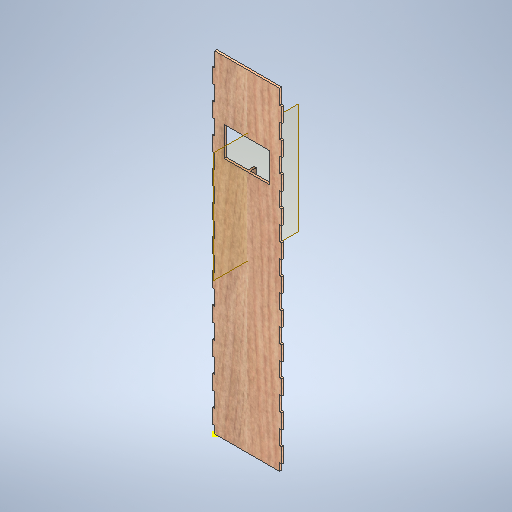
# Autodesk Inventor part: Part4 box
Saved by Autodesk Inventor 2025.3 (Build 293356000, 356)
## iProperties
Created: 2026-04-05
Part Number: Part4 box
Material: Wood (Birch)
Document SubType Name: Modeling
Designer: logien
Density: 0.55 g/cm^3
Appearance: Birch - Natural Polished
Author: logien
Autodesk Inventor part; units mm, degrees
ref_plane "YZ Plane" through (0, 0, 0) normal (1, 0, 0) x (0, 1, 0)
ref_plane "XZ Plane" through (0, 0, 0) normal (0, 1, 0) x (-1, 0, 0)
ref_plane "XY Plane" through (0, 0, 0) normal (0, 0, 1) x (1, 0, 0)
sketch "Sketch1" plane through (0, 0, 0) normal (0, 0, 1) x (1, 0, 0)
  line L0 (0, 0) -> (88, 0)
  line L1 (88, 0) -> (88, 10)
  line L2 (88, 10) -> (91, 10)
  line L3 (91, 10) -> (91, 30)
  line L4 (91, 30) -> (88, 30)
  line L5 (88, 30) -> (88, 50)
  line L6 (88, 50) -> (91, 50)
  line L7 (91, 50) -> (91, 70)
  line L8 (91, 70) -> (88, 70)
  line L9 (88, 70) -> (88, 90)
  line L10 (88, 90) -> (91, 90)
  line L11 (91, 90) -> (91, 110)
  line L12 (91, 110) -> (88, 110)
  line L13 (88, 110) -> (88, 130)
  line L14 (88, 130) -> (91, 130)
  line L15 (91, 130) -> (91, 150)
  line L16 (91, 150) -> (88, 150)
  line L17 (88, 150) -> (88, 170)
  line L18 (88, 170) -> (91, 170)
  line L19 (91, 170) -> (91, 190)
  line L20 (91, 190) -> (88, 190)
  line L21 (88, 190) -> (88, 210)
  line L22 (88, 210) -> (91, 210)
  line L23 (91, 210) -> (91, 230)
  line L24 (91, 230) -> (88, 230)
  line L25 (88, 230) -> (88, 250)
  line L26 (88, 250) -> (91, 250)
  line L27 (91, 250) -> (91, 270)
  line L28 (91, 270) -> (88, 270)
  line L29 (88, 270) -> (88, 290)
  line L30 (88, 290) -> (91, 290)
  line L31 (91, 290) -> (91, 310)
  line L32 (91, 310) -> (88, 310)
  line L33 (88, 310) -> (88, 330)
  line L34 (88, 330) -> (91, 330)
  line L35 (91, 330) -> (91, 350)
  line L36 (91, 350) -> (88, 350)
  line L37 (88, 350) -> (88, 370)
  line L38 (88, 370) -> (91, 370)
  line L39 (91, 370) -> (91, 390)
  line L40 (91, 390) -> (88, 390)
  line L41 (88, 390) -> (88, 410)
  line L42 (88, 410) -> (91, 410)
  line L43 (91, 410) -> (91, 430)
  line L44 (91, 430) -> (88, 430)
  line L45 (44, 0) -> (44, 110) construction
  line L46 (-3, 10) -> (-3, 30)
  line L47 (-3, 30) -> (0, 30)
  line L48 (0, 10) -> (-3, 10)
  line L49 (0, 50) -> (-3, 50)
  line L50 (-3, 50) -> (-3, 70)
  line L51 (0, 70) -> (0, 90)
  line L52 (0, 90) -> (-3, 90)
  line L53 (-3, 90) -> (-3, 110)
  line L54 (-3, 70) -> (0, 70)
  line L55 (-3, 110) -> (0, 110)
  line L56 (0, 110) -> (0, 130)
  line L57 (0, 130) -> (-3, 130)
  line L58 (-3, 130) -> (-3, 150)
  line L59 (-3, 170) -> (-3, 190)
  line L60 (0, 150) -> (0, 170)
  line L61 (0, 170) -> (-3, 170)
  line L62 (-3, 150) -> (0, 150)
  line L63 (0, 190) -> (0, 210)
  line L64 (-3, 190) -> (0, 190)
  line L65 (0, 210) -> (-3, 210)
  line L66 (-3, 210) -> (-3, 230)
  line L67 (-3, 230) -> (0, 230)
  line L68 (0, 230) -> (0, 250)
  line L69 (0, 250) -> (-3, 250)
  line L70 (-3, 250) -> (-3, 270)
  line L71 (-3, 270) -> (0, 270)
  line L72 (0, 270) -> (0, 290)
  line L73 (0, 290) -> (-3, 290)
  line L74 (-3, 290) -> (-3, 310)
  line L75 (-3, 310) -> (0, 310)
  line L76 (0, 310) -> (0, 330)
  line L77 (0, 350) -> (0, 370)
  line L78 (-3, 350) -> (0, 350)
  line L79 (-3, 330) -> (-3, 350)
  line L80 (0, 330) -> (-3, 330)
  line L81 (0, 370) -> (-3, 370)
  line L82 (-3, 370) -> (-3, 390)
  line L83 (-3, 390) -> (0, 390)
  line L84 (0, 390) -> (0, 410)
  line L85 (0, 410) -> (-3, 410)
  line L86 (-3, 410) -> (-3, 430)
  line L87 (-3, 430) -> (0, 430)
  line L88 (0, 430) -> (0, 450)
  line L89 (0, 450) -> (88, 450)
  line L90 (88, 430) -> (88, 450)
  line L91 (0, 50) -> (0, 30)
  line L92 (0, 10) -> (0, 0)
  point P0 (0, 0)
  dimension "d1" = 10
  dimension "d2" = 3
  dimension "d3" = 20
  dimension "d4" = 3
  dimension "d5" = 20
  dimension "d6" = 20
  dimension "d7" = 20
  dimension "d8" = 20
  dimension "d9" = 20
  dimension "d10" = 3
  dimension "d11" = 20
  dimension "d12" = 20
  dimension "d13" = 20
  dimension "d14" = 3
  dimension "d15" = 20
  dimension "d16" = 3
  dimension "d17" = 20
  dimension "d18" = 20
  dimension "d19" = 20
  dimension "d20" = 3
  dimension "d21" = 20
  dimension "d22" = 20
  dimension "d23" = 20
  dimension "d24" = 20
  dimension "d25" = 20
  dimension "d26" = 20
  dimension "d27" = 20
  dimension "d28" = 20
  dimension "d30" = 0
  dimension "d31" = 0
  dimension "d34" = 110
  dimension "d35" = 0
  dimension "d36" = 0
  dimension "d37" = 0
  dimension "d38" = 0
  dimension "d39" = 3
  dimension "d43" = 88
  dimension "d65" = 20
  constraints: 186 end point, 46 point on line, 44 symmetric about line, 26 perpendicular, 5 horizontal, 5 vertical, 1 midpoint, 1 parallel
  measures "d1" distance of L0.end L1.end
  measures "d2" distance of L1.end L2.end
  measures "d3" distance of L2.end L4.start
  measures "d4" distance of L4.start L5.start
  measures "d5" distance of L5.start L6.start
  measures "d6" distance of L7.start L8.start
  measures "d7" distance of L9.start L10.start
  measures "d8" distance of L10.end L11.end
  measures "d9" distance of L12.end L13.end
  measures "d10" distance of L13.end L14.end
  measures "d11" distance of L14.end L15.end
  measures "d12" distance of L16.end L17.end
  measures "d13" distance of L18.end L19.end
  measures "d14" distance of L19.end L20.end
  measures "d15" distance of L20.end L22.start
  measures "d16" distance of L22.start L22.end
  measures "d17" distance of L22.end L24.start
  measures "d18" distance of L24.end L26.start
  measures "d19" distance of L26.end L27.end
  measures "d20" distance of L27.end L28.end
  measures "d21" distance of L28.end L30.start
  measures "d22" distance of L30.end L32.start
  measures "d23" distance of L32.end L33.end
  measures "d24" distance of L34.end L36.start
  measures "d25" distance of L36.end L37.end
  measures "d26" distance of L38.end L39.end
  measures "d27" distance of L40.end L41.end
  measures "d28" distance of L42.end L43.end
  measures "d30" distance of L0.start point (0, 0)
  measures "d31" distance of L0.start point (0, 0)
  measures "d34" distance of L45.start L45.end
  measures "d35" distance between parallel lines of L35 L39
  measures "d36" distance between parallel lines of L39 L19
  measures "d37" distance between parallel lines of L39 L15
  measures "d38" distance between parallel lines of L39 L3
  measures "d39" distance between parallel lines of L41 L39
  measures "d43" distance of L0.start L0.end
  measures "d65" distance of L87.end L88.end
extrude "Extrusion1" add sketch "Sketch1" along normal blind 3
sketch "Sketch4" plane through (0, 0, 0) normal (0, 0, -1) x (-1, 0, 0)
  line L0 (-98.5, 430) -> (-44, 430)
  line L1 (-91, 430) -> (3, 430) projected
  line L2 (-44.5, 330) -> (-75, 330)
  line L3 (-75, 350) -> (-75, 0) projected
  line L4 (-75, 330) -> (-75, 370)
  line L5 (-75, 370) -> (-43, 370)
  line L6 (-43, 370) -> (-13, 370)
  line L7 (-13, 370) -> (-13, 330)
  line L8 (-13, 330) -> (-44.5, 330)
  line L9 (0, 370) -> (0, 350) projected
  point P0 (0, 0)
  dimension "d55" = 30
  dimension "d58" = 60
  dimension "d59" = 40
  dimension "d61" = 30.5
  dimension "d62" = 0
  dimension "d63" = 80
  dimension "d64" = 23.5
  dimension "d66" = 13
  constraints: 14 end point, 2 point on line, 1 collinear, 1 horizontal, 1 midpoint, 1 parallel, 1 perpendicular, 1 vertical
  measures "d55" distance of L5.end L6.end
  measures "d58" distance between parallel lines of L0 L5
  measures "d59" distance between parallel lines of L2 L5
  measures "d61" distance from line of L2.start L3
  measures "d62" distance from line of point (-75, 350) L3
  measures "d63" distance from line of point (-75, 350) L1
  measures "d64" distance from line of L0.start L3
  measures "d66" distance between parallel lines of L7 L9
extrude "Extrusion4" cut sketch "Sketch4" against normal blind 19
sketch "Sketch5" plane through (0, 0, 3) normal (0, 0, 1) x (1, 0, 0)
  point P0 (0, 0)
sketch "Sketch6" plane through (0, 0, 0) normal (0, 0, -1) x (-1, 0, 0)
  line L0 (0, 0) -> (-88, 0) projected
  line L1 (-44, 0) -> (-44, 330)
  line L2 (-75, 330) -> (-13, 330) projected
  line L3 (-44, 0) -> (-42.5, 0)
  line L4 (-42.5, 0) -> (-42.5, 330)
  line L5 (-44, 330) -> (-45.5, 330)
  line L6 (-45.5, 330) -> (-45.5, 0)
  line L7 (-44, 0) -> (-45.5, 0)
  dimension "d67" = 1.5
  dimension "d68" = 1.5
  constraints: 12 end point, 4 point on line, 3 perpendicular, 2 midpoint
  measures "d67" distance of L1.start L3.end
  measures "d68" distance of L1.end L5.end
extrude "Extrusion5" add sketch "Sketch6" along normal blind 8
ref_plane "Work Plane1" through (44, 430, 0) normal (1, 0, 0) x (0, 0, -1)
body "Solid1"
